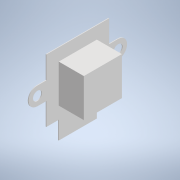
# Autodesk Inventor part: ov13855
Saved by Autodesk Inventor 2022 (Build 260153000, 153)
## iProperties
Created: 2024-12-21
Part Number: ov13855
Material: Типовые
Document SubType Name: Modeling
Designer: Andrey
Density: 1 g/cm^3
Appearance: По умолчанию
Author: Andrey
Autodesk Inventor part; units mm, degrees
ref_plane "YZ Plane" through (0, 0, 0) normal (1, 0, 0) x (0, 1, 0)
ref_plane "XZ Plane" through (0, 0, 0) normal (0, 1, 0) x (-1, 0, 0)
ref_plane "XY Plane" through (0, 0, 0) normal (0, 0, 1) x (1, 0, 0)
sketch "Эскиз1" plane through (0, 0, 0) normal (1, 0, 0) x (0, 1, 0)
  line L0 (-7, 7) -> (7, 7)
  line L1 (7, 7) -> (7, -7)
  line L2 (7, -7) -> (-7, -7)
  line L3 (-7, -7) -> (-7, 7)
  line L4 (-7, 7) -> (7, -7) construction
  line L5 (7, 7) -> (-7, -7) construction
  line L6 (0, 9) -> (0, -9)
  circle A0 centre (0, -9) radius 2
  circle A1 centre (0, 9) radius 2
  line L7 (2, 9) -> (2, -9)
  line L8 (-2, -9) -> (-2, 9)
  line L9 (4.25, 4.25) -> (-4.25, 4.25)
  line L10 (-4.25, 4.25) -> (-4.25, -4.25)
  line L11 (-4.25, -4.25) -> (4.25, -4.25)
  line L12 (4.25, -4.25) -> (4.25, 4.25)
  line L13 (4.25, 4.25) -> (-4.25, -4.25) construction
  line L14 (-4.25, 4.25) -> (4.25, -4.25) construction
  line L15 (-7, 4.25) -> (-11, 4.25)
  line L16 (-11, 4.25) -> (-11, -4.25)
  line L17 (-11, -4.25) -> (-7, -4.25)
  line L18 (-7, -4.25) -> (-7, 4.25)
  circle A2 centre (0, 9) radius 1
  circle A3 centre (0, -9) radius 1
  point P0 (0, 0)
  point P1 (0, 0)
  point P2 (2, -7)
  point P3 (2, 7)
  point P4 (-2, 7)
  point P5 (-2, -7)
  dimension "d0" = 14
  dimension "d1" = 14
  dimension "d2" = 18
  dimension "d3" = 8.5
  dimension "d4" = 8.5
  dimension "d5" = 4
  dimension "d6" = 2
  dimension "d7" = 2
  constraints: 38 end point, 6 midpoint, 6 parallel, 6 tangent, 4 centre point, 4 coincident, 4 point on circle, 3 horizontal, 3 perpendicular, 2 collinear, 1 point on line, 1 vertical
  measures "d0" distance of L1.end L2.end
  measures "d1" distance of L0.end L1.end
  measures "d2" distance of L6.start L6.end
  measures "d3" distance of L11.end L10.end
  measures "d4" distance of L10.end L9.end
  measures "d5" distance of L17.end L16.end
  measures "d6" diameter of A2
  measures "d7" diameter of A3
extrude "Выдавливание1" add sketch "Эскиз1" along normal blind 0.15
sketch "Эскиз2" plane through (0, 0, 0) normal (-1, 0, 0) x (0, 0, 1)
  line L0 (-4.25, 4.25) -> (4.25, 4.25)
  line L1 (4.25, 4.25) -> (4.25, -4.25)
  line L2 (4.25, -4.25) -> (-4.25, -4.25)
  line L3 (-4.25, -4.25) -> (-4.25, 4.25)
  line L4 (-4.25, 4.25) -> (4.25, -4.25) construction
  line L5 (4.25, 4.25) -> (-4.25, -4.25) construction
  point P0 (0, 0)
  dimension "d10" = 8.5
  dimension "d11" = 8.5
  constraints: 12 end point, 2 midpoint, 2 parallel, 1 horizontal, 1 perpendicular
  measures "d10" distance of L1.end L2.end
  measures "d11" distance of L0.end L1.end
extrude "Выдавливание2" add sketch "Эскиз2" against normal blind 5.75
